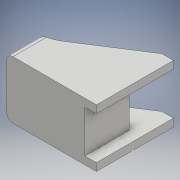
# Autodesk Inventor part: anchorage
Saved by Autodesk Inventor 2017 (Build 210142000, 142)
## iProperties
Part Number: anchorage
Material: 一般
Document SubType Name: Modeling
Designer: 3890237626
Density: 1 g/cm^3
Appearance: 既定
Author: 3890237626
Autodesk Inventor part; units mm, degrees
ref_plane "YZ Plane" through (0, 0, 0) normal (1, 0, 0) x (0, 1, 0)
ref_plane "XZ Plane" through (0, 0, 0) normal (0, 1, 0) x (-1, 0, 0)
ref_plane "XY Plane" through (0, 0, 0) normal (0, 0, 1) x (1, 0, 0)
sketch "スケッチ1" plane through (0, 0, 0) normal (0, 0, 1) x (1, 0, 0)
  line L0 (-174813.9436, -2410.1862) -> (-174813.9436, -27910.1862)
  line L1 (-174813.9436, -27910.1862) -> (-104813.9436, -27910.1862)
  line L2 (-104813.9436, -27910.1862) -> (-104813.9436, 32089.8138)
  line L3 (-104813.9436, 32089.8138) -> (-113813.9436, 32089.8138)
  line L4 (-113813.9436, 32089.8138) -> (-159813.9436, 2589.8138)
  spline S0 degree 3 poles (-159813.9436, 2589.8138) (-164318.6072, -299.0466) (-169408.2494, -2410.1862) (-174813.9436, -2410.1862) knots 0 0 0 0 1 1 1 1
  point P0 (0, 0)
  dimension "d0" = 70000
  dimension "d1" = 25500
  dimension "d2" = 5000
  dimension "d3" = 9000
  dimension "d4" = 15000
  dimension "d5" = 60000
  constraints: 10 end point, 2 perpendicular, 2 vertical, 1 horizontal, 3 other
  measures "d0" distance of L0.end L1.end
  measures "d1" distance of L0.start L0.end
  measures "d2" vertical distance of L0.start L4.end
  measures "d3" distance of L2.end L3.end
  measures "d4" horizontal distance of L0.start L4.end
  measures "d5" distance of L1.end L2.end
extrude "押し出し1" add sketch "スケッチ1" along normal blind 45000
sketch "スケッチ2" plane through (-104813.9436, -27910.1862, 0) normal (1, 0, 0) x (0, 0, -1)
  point P0 (0, 27910.1862)
sketch "スケッチ3" plane through (-113813.9436, 32089.8138, 0) normal (0, 1, 0) x (1, 0, 0)
  line L0 (9000, 0) -> (0, 0) projected
  line L1 (0, 0) -> (0, -45000) projected
  line L2 (9000, -45000) -> (0, -45000) projected
  line L3 (9000, 0) -> (9000, -45000) projected
  line L4 (9000, -39000) -> (0, -39000)
  line L5 (0, -39000) -> (0, -6000)
  line L6 (0, -6000) -> (9000, -6000)
  line L7 (9000, -6000) -> (9000, -39000)
  point P0 (113813.9436, 0)
  dimension "d8" = 33000
  dimension "d9" = 6000
  constraints: 8 end point, 2 parallel, 2 point on line, 1 horizontal, 1 perpendicular
  measures "d8" distance of L6.end L4.start
  measures "d9" distance of L4.start L2.start
extrude "押し出し2" cut sketch "スケッチ3" against normal blind 60000 contours L3 L4 L1 L6
sketch "スケッチ4" plane through (-104813.9436, -27910.1862, 0) normal (1, 0, 0) x (0, 0, -1)
  line L0 (-6000, 60000) -> (-6000, 0) projected
  line L1 (0, 0) -> (-6000, 0) projected
  line L2 (0, 0) -> (0, 60000) projected
  line L3 (0, 60000) -> (-6000, 60000) projected
  line L4 (-6000, 60000) -> (-39000, 60000) projected
  line L5 (-39000, 60000) -> (-39000, 0) projected
  line L6 (-6000, 0) -> (-39000, 0) projected
  line L7 (-6000, 60000) -> (-6000, 0) projected
  line L8 (-39000, 0) -> (-39000, 60000) projected
  line L9 (-39000, 60000) -> (-45000, 60000) projected
  line L10 (-45000, 0) -> (-45000, 60000) projected
  line L11 (-39000, 0) -> (-45000, 0) projected
  line L12 (-6000, 60000) -> (-39000, 60000)
  line L13 (-39000, 60000) -> (-39000, 34500)
  line L14 (-39000, 34500) -> (-6000, 34500)
  line L15 (-6000, 34500) -> (-6000, 60000)
  point P0 (0, 27910.1862)
  dimension "d12" = 34500
  constraints: 8 end point, 2 parallel, 1 horizontal, 1 perpendicular, 1 point on line
  measures "d12" distance between parallel lines of L6 L14
extrude "押し出し3" cut sketch "スケッチ4" against normal blind 60000 contours L0 L14 L5 L4
sketch "スケッチ5" plane through (-174813.9436, -27910.1862, 0) normal (0, -1, 0) x (1, 0, 0)
  line L0 (70000, 6000) -> (61000, 6000) projected
  line L1 (61000, 6000) -> (61000, 39000) projected
  line L2 (61000, 39000) -> (70000, 39000) projected
  line L3 (70000, 39000) -> (70000, 45000) projected
  line L4 (0, 45000) -> (70000, 45000) projected
  line L5 (0, 0) -> (0, 45000) projected
  line L6 (0, 0) -> (70000, 0) projected
  line L7 (70000, 0) -> (70000, 6000) projected
  arc A0 (0, 5000) -> (5000, 0) centre (5000, 5000) ccw
  arc A1 (5000, 45000) -> (0, 40000) centre (5000, 40000) ccw
  point P0 (174813.9436, 0)
  dimension "d15" = 5000
  constraints: 4 point on circle, 4 point on line, 4 tangent, 2 centre point, 1 equal radius
  measures "d15" radius of A0
extrude "押し出し4" cut sketch "スケッチ5" against normal blind 100000 contours L6 L5 A0 | L5 L4 A1
